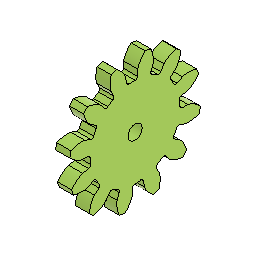
03 Engranaje (para servomotor) (Autodesk Fusion 360 design; units mm, degrees)
Autodesk Fusion 360 part; units mm, degrees
(part 1 of 2)
sketch "Boceto1" plane through (0, 0, 0) normal (0, 0, 1) x (1, 0, 0)
  circle A0 centre (0, 0) radius 9.5
  circle A1 centre (0, 0) radius 0.5
extrude "Extruir1" add sketch "Boceto1" along normal blind 3
sketch "Boceto2" plane through (0, 0, 0) normal (0, 0, 1) x (1, 0, 0)
  spline S0 degree 5 poles (11.1567, -1.6383) (11.1647, -1.6395) (11.1807, -1.6416) (11.2048, -1.6439) (11.237, -1.6456) (11.2774, -1.6458) (11.318, -1.6445) (11.3587, -1.6423) (11.3994, -1.6396) (11.4401, -1.6366) (11.4809, -1.6333) (11.5218, -1.6295) (11.5626, -1.625) (11.6035, -1.6199) (11.6445, -1.614) (11.6854, -1.6075) (11.7264, -1.6005) (11.7674, -1.5929) (11.8084, -1.585) (11.8494, -1.5766) (11.8905, -1.5678) (11.9315, -1.5587) (11.9725, -1.5491) (12.0135, -1.539) (12.0545, -1.5285) (12.0956, -1.5175) (12.1366, -1.5062) (12.1776, -1.4944) (12.2186, -1.4823) (12.2595, -1.4698) (12.3005, -1.4569) (12.3414, -1.4437) (12.3824, -1.4301) (12.4233, -1.4161) (12.4641, -1.4018) (12.505, -1.3871) (12.5458, -1.372) (12.5866, -1.3566) (12.6274, -1.3409) (12.6681, -1.3248) (12.7088, -1.3084) (12.7495, -1.2917) (12.7902, -1.2746) (12.8308, -1.2572) (12.8713, -1.2395) (12.9119, -1.2215) (12.9523, -1.2031) (12.9928, -1.1844) (13.0332, -1.1654) (13.0735, -1.1461) (13.1138, -1.1265) (13.1541, -1.1066) (13.1943, -1.0863) (13.2345, -1.0658) (13.2746, -1.045) (13.3146, -1.0239) (13.3546, -1.0024) (13.3946, -0.9807) (13.4344, -0.9587) (13.4743, -0.9364) (13.514, -0.9138) (13.5538, -0.8909) (13.5934, -0.8678) (13.633, -0.8443) (13.6725, -0.8206) (13.712, -0.7966) (13.7514, -0.7723) (13.7907, -0.7477) (13.8299, -0.7229) (13.8691, -0.6978) (13.9082, -0.6724) (13.9395, -0.6518) (13.9629, -0.6363) (13.9784, -0.6259) (13.9862, -0.6207) knots 0 0 0 0 0 0 0.01428571 0.02857143 0.04285714 0.05714286 0.07142857 0.08571429 0.1 0.11428571 0.12857143 0.14285714 0.15714286 0.17142857 0.18571429 0.2 0.21428571 0.22857143 0.24285714 0.25714286 0.27142857 0.28571429 0.3 0.31428571 0.32857143 0.34285714 0.35714286 0.37142857 0.38571429 0.4 0.41428571 0.42857143 0.44285714 0.45714286 0.47142857 0.48571429 0.5 0.51428571 0.52857143 0.54285714 0.55714286 0.57142857 0.58571429 0.6 0.61428571 0.62857143 0.64285714 0.65714286 0.67142857 0.68571429 0.7 0.71428571 0.72857143 0.74285714 0.75714286 0.77142857 0.78571429 0.8 0.81428571 0.82857143 0.84285714 0.85714286 0.87142857 0.88571429 0.9 0.91428571 0.92857143 0.94285714 0.95714286 0.97142857 0.98571429 1 1 1 1 1 1
  spline S1 degree 5 poles (11.1567, 1.6383) (11.1647, 1.6395) (11.1807, 1.6416) (11.2048, 1.6439) (11.237, 1.6456) (11.2774, 1.6458) (11.318, 1.6445) (11.3587, 1.6423) (11.3994, 1.6396) (11.4401, 1.6366) (11.4809, 1.6333) (11.5218, 1.6295) (11.5626, 1.625) (11.6035, 1.6199) (11.6445, 1.614) (11.6854, 1.6075) (11.7264, 1.6005) (11.7674, 1.5929) (11.8084, 1.585) (11.8494, 1.5766) (11.8905, 1.5678) (11.9315, 1.5587) (11.9725, 1.5491) (12.0135, 1.539) (12.0545, 1.5285) (12.0956, 1.5175) (12.1366, 1.5062) (12.1776, 1.4944) (12.2186, 1.4823) (12.2595, 1.4698) (12.3005, 1.4569) (12.3414, 1.4437) (12.3824, 1.4301) (12.4233, 1.4161) (12.4641, 1.4018) (12.505, 1.3871) (12.5458, 1.372) (12.5866, 1.3566) (12.6274, 1.3409) (12.6681, 1.3248) (12.7088, 1.3084) (12.7495, 1.2917) (12.7902, 1.2746) (12.8308, 1.2572) (12.8713, 1.2395) (12.9119, 1.2215) (12.9523, 1.2031) (12.9928, 1.1844) (13.0332, 1.1654) (13.0735, 1.1461) (13.1138, 1.1265) (13.1541, 1.1066) (13.1943, 1.0863) (13.2345, 1.0658) (13.2746, 1.045) (13.3146, 1.0239) (13.3546, 1.0024) (13.3946, 0.9807) (13.4344, 0.9587) (13.4743, 0.9364) (13.514, 0.9138) (13.5538, 0.8909) (13.5934, 0.8678) (13.633, 0.8443) (13.6725, 0.8206) (13.712, 0.7966) (13.7514, 0.7723) (13.7907, 0.7477) (13.8299, 0.7229) (13.8691, 0.6978) (13.9082, 0.6724) (13.9395, 0.6518) (13.9629, 0.6363) (13.9784, 0.6259) (13.9862, 0.6207) knots 0 0 0 0 0 0 0.01428571 0.02857143 0.04285714 0.05714286 0.07142857 0.08571429 0.1 0.11428571 0.12857143 0.14285714 0.15714286 0.17142857 0.18571429 0.2 0.21428571 0.22857143 0.24285714 0.25714286 0.27142857 0.28571429 0.3 0.31428571 0.32857143 0.34285714 0.35714286 0.37142857 0.38571429 0.4 0.41428571 0.42857143 0.44285714 0.45714286 0.47142857 0.48571429 0.5 0.51428571 0.52857143 0.54285714 0.55714286 0.57142857 0.58571429 0.6 0.61428571 0.62857143 0.64285714 0.65714286 0.67142857 0.68571429 0.7 0.71428571 0.72857143 0.74285714 0.75714286 0.77142857 0.78571429 0.8 0.81428571 0.82857143 0.84285714 0.85714286 0.87142857 0.88571429 0.9 0.91428571 0.92857143 0.94285714 0.95714286 0.97142857 0.98571429 1 1 1 1 1 1
  arc A0 (13.9862, -0.6207) -> (13.9862, 0.6207) centre (0, 0) ccw
  line L0 (9.3893, -1.3802) -> (11.1567, -1.6383)
  line L1 (9.3893, 1.3802) -> (11.1567, 1.6383)
  line L2 (9.3893, -1.3802) -> (9.3893, 1.3802)
  point P0 (11.3527, -1.6425)
  point P1 (11.5515, -1.6261)
  point P2 (11.7521, -1.5957)
  point P3 (11.954, -1.5533)
  point P4 (12.1568, -1.5003)
  point P5 (12.3603, -1.4374)
  point P6 (12.5642, -1.3651)
  point P7 (12.7683, -1.2838)
  point P8 (12.9724, -1.1938)
  point P9 (13.1764, -1.0953)
  point P10 (13.3799, -0.9887)
  point P11 (13.5828, -0.8739)
  point P12 (13.785, -0.7512)
  point P13 (11.3527, 1.6425)
  point P14 (11.5515, 1.6261)
  point P15 (11.7521, 1.5957)
  point P16 (11.954, 1.5533)
  point P17 (12.1568, 1.5003)
  point P18 (12.3603, 1.4374)
  point P19 (12.5642, 1.3651)
  point P20 (12.7683, 1.2838)
  point P21 (12.9724, 1.1938)
  point P22 (13.1764, 1.0953)
  point P23 (13.3799, 0.9887)
  point P24 (13.5828, 0.8739)
  point P25 (13.785, 0.7512)
extrude "Extruir2" add sketch "Boceto2" along normal blind 3
fillet "Empalme1" radius 0.5 2 edges at (9.399, -1.3817, 1.5) (9.399, 1.3817, 1.5)
pattern_circular "Patrón C1" count 12 over 360 about axis through (0, 0, 0) along (0, 0, 1) of "Extruir2", "Empalme1"
sketch "Boceto3" plane through (0, 0, 0) normal (0, 0, 1) x (1, 0, 0)
  circle A0 centre (0, 0) radius 12 construction
move_body "Desplazar1" bodies 1 to x (0.660356, 0.750952, 0) y (-0.750952, 0.660356, 0) z (0, 0, 1) at (0, 0, 0)
move_body "Desplazar2" bodies 1 to x (0, 0, -1) y (0, 1, 0) z (1, 0, 0) at (0, 0, 0)
move_body "Desplazar3" bodies 1 to x (1, 0, 0) y (0, 1, 0) z (0, 0, 1) at (0, 47.5478, 13.9934)
sketch "Boceto4" plane through (0, 0, 0) normal (-1, 0, 0) x (0, -1, 0)
  circle A0 centre (-47.5478, 13.9934) radius 0.5
  arc A1 (-47.0309, 4.0198) -> (-47.5311, 4.4934) centre (-47.5302, 3.9934) ccw
  line L0 (-47.0309, 4.0198) -> (-46.963, 2.7323)
  spline S0 degree 5 poles (-46.963, 2.7323) (-46.9625, 2.7242) (-46.9614, 2.7081) (-46.959, 2.684) (-46.9543, 2.6521) (-46.9465, 2.6124) (-46.9373, 2.5729) (-46.9272, 2.5335) (-46.9166, 2.494) (-46.9056, 2.4547) (-46.8943, 2.4153) (-46.8826, 2.3761) (-46.8702, 2.3369) (-46.8571, 2.2978) (-46.8433, 2.2588) (-46.8289, 2.2199) (-46.8139, 2.1811) (-46.7985, 2.1424) (-46.7826, 2.1037) (-46.7664, 2.0651) (-46.7497, 2.0266) (-46.7327, 1.9882) (-46.7152, 1.9499) (-46.6973, 1.9116) (-46.6789, 1.8735) (-46.6601, 1.8354) (-46.6409, 1.7974) (-46.6213, 1.7595) (-46.6014, 1.7217) (-46.5811, 1.684) (-46.5604, 1.6464) (-46.5394, 1.6088) (-46.5181, 1.5714) (-46.4963, 1.534) (-46.4742, 1.4967) (-46.4518, 1.4596) (-46.429, 1.4225) (-46.4059, 1.3855) (-46.3825, 1.3486) (-46.3587, 1.3118) (-46.3346, 1.2751) (-46.3102, 1.2385) (-46.2855, 1.202) (-46.2605, 1.1656) (-46.2351, 1.1294) (-46.2095, 1.0932) (-46.1835, 1.0571) (-46.1573, 1.0211) (-46.1307, 0.9852) (-46.1039, 0.9494) (-46.0767, 0.9138) (-46.0493, 0.8782) (-46.0215, 0.8428) (-45.9935, 0.8074) (-45.9652, 0.7722) (-45.9366, 0.7371) (-45.9078, 0.702) (-45.8786, 0.6671) (-45.8492, 0.6324) (-45.8195, 0.5977) (-45.7896, 0.5631) (-45.7593, 0.5287) (-45.7288, 0.4944) (-45.698, 0.4601) (-45.667, 0.4261) (-45.6357, 0.3921) (-45.6042, 0.3582) (-45.5724, 0.3245) (-45.5403, 0.2909) (-45.508, 0.2574) (-45.4754, 0.224) (-45.4491, 0.1974) (-45.4293, 0.1776) (-45.416, 0.1643) (-45.4094, 0.1577) knots 0 0 0 0 0 0 0.01428571 0.02857143 0.04285714 0.05714286 0.07142857 0.08571429 0.1 0.11428571 0.12857143 0.14285714 0.15714286 0.17142857 0.18571429 0.2 0.21428571 0.22857143 0.24285714 0.25714286 0.27142857 0.28571429 0.3 0.31428571 0.32857143 0.34285714 0.35714286 0.37142857 0.38571429 0.4 0.41428571 0.42857143 0.44285714 0.45714286 0.47142857 0.48571429 0.5 0.51428571 0.52857143 0.54285714 0.55714286 0.57142857 0.58571429 0.6 0.61428571 0.62857143 0.64285714 0.65714286 0.67142857 0.68571429 0.7 0.71428571 0.72857143 0.74285714 0.75714286 0.77142857 0.78571429 0.8 0.81428571 0.82857143 0.84285714 0.85714286 0.87142857 0.88571429 0.9 0.91428571 0.92857143 0.94285714 0.95714286 0.97142857 0.98571429 1 1 1 1 1 1
  arc A2 (-45.4094, 0.1577) -> (-44.1922, 0.4015) centre (-47.5478, 13.9934) ccw
  spline S1 degree 5 poles (-43.7502, 3.3759) (-43.7474, 3.3682) (-43.7423, 3.3529) (-43.7352, 3.3298) (-43.7272, 3.2985) (-43.7191, 3.2589) (-43.7124, 3.2189) (-43.7066, 3.1786) (-43.7012, 3.1381) (-43.6961, 3.0976) (-43.6914, 3.0569) (-43.6871, 3.0161) (-43.6834, 2.9752) (-43.6805, 2.9341) (-43.6782, 2.8928) (-43.6765, 2.8513) (-43.6754, 2.8098) (-43.6747, 2.7681) (-43.6745, 2.7263) (-43.6746, 2.6845) (-43.6751, 2.6425) (-43.6761, 2.6005) (-43.6774, 2.5584) (-43.6792, 2.5162) (-43.6815, 2.4739) (-43.6842, 2.4315) (-43.6873, 2.3891) (-43.6907, 2.3466) (-43.6946, 2.304) (-43.6988, 2.2614) (-43.7033, 2.2187) (-43.7083, 2.1759) (-43.7136, 2.1331) (-43.7192, 2.0903) (-43.7253, 2.0474) (-43.7317, 2.0044) (-43.7384, 1.9614) (-43.7455, 1.9184) (-43.7529, 1.8753) (-43.7606, 1.8322) (-43.7687, 1.7891) (-43.7772, 1.7459) (-43.7859, 1.7027) (-43.795, 1.6595) (-43.8044, 1.6163) (-43.8142, 1.573) (-43.8242, 1.5297) (-43.8346, 1.4864) (-43.8453, 1.443) (-43.8563, 1.3997) (-43.8676, 1.3563) (-43.8792, 1.3129) (-43.8912, 1.2695) (-43.9034, 1.2261) (-43.9159, 1.1827) (-43.9288, 1.1392) (-43.9419, 1.0958) (-43.9554, 1.0524) (-43.9691, 1.009) (-43.9832, 0.9655) (-43.9975, 0.9221) (-44.0122, 0.8787) (-44.0271, 0.8352) (-44.0423, 0.7918) (-44.0578, 0.7484) (-44.0736, 0.705) (-44.0897, 0.6616) (-44.1061, 0.6182) (-44.1227, 0.5748) (-44.1396, 0.5315) (-44.1569, 0.4882) (-44.1708, 0.4535) (-44.1815, 0.4275) (-44.1886, 0.4102) (-44.1922, 0.4015) knots 0 0 0 0 0 0 0.01428571 0.02857143 0.04285714 0.05714286 0.07142857 0.08571429 0.1 0.11428571 0.12857143 0.14285714 0.15714286 0.17142857 0.18571429 0.2 0.21428571 0.22857143 0.24285714 0.25714286 0.27142857 0.28571429 0.3 0.31428571 0.32857143 0.34285714 0.35714286 0.37142857 0.38571429 0.4 0.41428571 0.42857143 0.44285714 0.45714286 0.47142857 0.48571429 0.5 0.51428571 0.52857143 0.54285714 0.55714286 0.57142857 0.58571429 0.6 0.61428571 0.62857143 0.64285714 0.65714286 0.67142857 0.68571429 0.7 0.71428571 0.72857143 0.74285714 0.75714286 0.77142857 0.78571429 0.8 0.81428571 0.82857143 0.84285714 0.85714286 0.87142857 0.88571429 0.9 0.91428571 0.92857143 0.94285714 0.95714286 0.97142857 0.98571429 1 1 1 1 1 1
  line L1 (-43.7502, 3.3759) -> (-44.1834, 4.5902)
  arc A3 (-43.9042, 5.2199) -> (-44.1834, 4.5902) centre (-43.7125, 4.7582) ccw
  arc A4 (-43.9042, 5.2199) -> (-42.7833, 5.7746) centre (-47.5478, 13.9934) ccw
  arc A5 (-42.1133, 5.6145) -> (-42.7833, 5.7746) centre (-42.5325, 5.342) ccw
  line L2 (-42.1133, 5.6145) -> (-41.4107, 4.5334)
  spline S2 degree 5 poles (-41.4107, 4.5334) (-41.4063, 4.5267) (-41.3973, 4.5133) (-41.3832, 4.4936) (-41.3632, 4.4683) (-41.3366, 4.4378) (-41.3088, 4.4082) (-41.2803, 4.3791) (-41.2515, 4.3503) (-41.2223, 4.3217) (-41.1928, 4.2933) (-41.163, 4.2651) (-41.1327, 4.2374) (-41.1018, 4.21) (-41.0704, 4.1832) (-41.0385, 4.1567) (-41.0061, 4.1306) (-40.9733, 4.1048) (-40.9403, 4.0792) (-40.9069, 4.0539) (-40.8733, 4.0289) (-40.8393, 4.0042) (-40.805, 3.9797) (-40.7703, 3.9556) (-40.7353, 3.9317) (-40.7, 3.9081) (-40.6644, 3.8848) (-40.6285, 3.8618) (-40.5923, 3.839) (-40.5559, 3.8165) (-40.5192, 3.7942) (-40.4822, 3.7722) (-40.445, 3.7505) (-40.4075, 3.729) (-40.3697, 3.7078) (-40.3317, 3.6868) (-40.2934, 3.6661) (-40.2549, 3.6456) (-40.2162, 3.6254) (-40.1772, 3.6054) (-40.138, 3.5857) (-40.0986, 3.5662) (-40.0589, 3.5469) (-40.0191, 3.5279) (-39.979, 3.5092) (-39.9387, 3.4906) (-39.8981, 3.4724) (-39.8574, 3.4543) (-39.8165, 3.4365) (-39.7753, 3.419) (-39.734, 3.4017) (-39.6924, 3.3846) (-39.6507, 3.3678) (-39.6087, 3.3512) (-39.5666, 3.3348) (-39.5243, 3.3187) (-39.4818, 3.3028) (-39.4391, 3.2871) (-39.3962, 3.2717) (-39.3532, 3.2565) (-39.31, 3.2416) (-39.2666, 3.2269) (-39.223, 3.2124) (-39.1792, 3.1981) (-39.1353, 3.1841) (-39.0912, 3.1704) (-39.047, 3.1568) (-39.0026, 3.1435) (-38.958, 3.1304) (-38.9132, 3.1176) (-38.8683, 3.105) (-38.8323, 3.0951) (-38.8052, 3.0878) (-38.7871, 3.083) (-38.778, 3.0806) knots 0 0 0 0 0 0 0.01428571 0.02857143 0.04285714 0.05714286 0.07142857 0.08571429 0.1 0.11428571 0.12857143 0.14285714 0.15714286 0.17142857 0.18571429 0.2 0.21428571 0.22857143 0.24285714 0.25714286 0.27142857 0.28571429 0.3 0.31428571 0.32857143 0.34285714 0.35714286 0.37142857 0.38571429 0.4 0.41428571 0.42857143 0.44285714 0.45714286 0.47142857 0.48571429 0.5 0.51428571 0.52857143 0.54285714 0.55714286 0.57142857 0.58571429 0.6 0.61428571 0.62857143 0.64285714 0.65714286 0.67142857 0.68571429 0.7 0.71428571 0.72857143 0.74285714 0.75714286 0.77142857 0.78571429 0.8 0.81428571 0.82857143 0.84285714 0.85714286 0.87142857 0.88571429 0.9 0.91428571 0.92857143 0.94285714 0.95714286 0.97142857 0.98571429 1 1 1 1 1 1
  arc A6 (-38.778, 3.0806) -> (-37.8458, 3.9003) centre (-47.5478, 13.9934) ccw
  spline S3 degree 5 poles (-38.9502, 6.6972) (-38.944, 6.6919) (-38.9319, 6.6813) (-38.9142, 6.6648) (-38.8916, 6.6417) (-38.8648, 6.6114) (-38.839, 6.5801) (-38.8138, 6.5481) (-38.7889, 6.5158) (-38.7642, 6.4832) (-38.7398, 6.4503) (-38.7157, 6.4172) (-38.6921, 6.3835) (-38.6689, 6.3494) (-38.6463, 6.3148) (-38.6241, 6.2798) (-38.6023, 6.2443) (-38.5809, 6.2086) (-38.5598, 6.1725) (-38.539, 6.1362) (-38.5185, 6.0996) (-38.4983, 6.0627) (-38.4784, 6.0256) (-38.4589, 5.9881) (-38.4397, 5.9504) (-38.4209, 5.9123) (-38.4023, 5.874) (-38.384, 5.8355) (-38.3661, 5.7967) (-38.3484, 5.7577) (-38.331, 5.7184) (-38.3139, 5.6789) (-38.2971, 5.6392) (-38.2806, 5.5993) (-38.2644, 5.5591) (-38.2484, 5.5187) (-38.2328, 5.4781) (-38.2174, 5.4373) (-38.2023, 5.3963) (-38.1874, 5.3551) (-38.1729, 5.3137) (-38.1586, 5.2721) (-38.1446, 5.2303) (-38.1308, 5.1884) (-38.1174, 5.1462) (-38.1041, 5.1038) (-38.0912, 5.0613) (-38.0785, 5.0186) (-38.0661, 4.9757) (-38.054, 4.9327) (-38.0421, 4.8895) (-38.0305, 4.8461) (-38.0191, 4.8025) (-38.008, 4.7588) (-37.9971, 4.7149) (-37.9866, 4.6709) (-37.9762, 4.6267) (-37.9662, 4.5824) (-37.9564, 4.5379) (-37.9468, 4.4932) (-37.9375, 4.4485) (-37.9285, 4.4035) (-37.9197, 4.3585) (-37.9111, 4.3132) (-37.9029, 4.2679) (-37.8948, 4.2224) (-37.8871, 4.1768) (-37.8796, 4.131) (-37.8723, 4.0852) (-37.8653, 4.0391) (-37.8585, 3.993) (-37.8533, 3.956) (-37.8495, 3.9282) (-37.847, 3.9096) (-37.8458, 3.9003) knots 0 0 0 0 0 0 0.01428571 0.02857143 0.04285714 0.05714286 0.07142857 0.08571429 0.1 0.11428571 0.12857143 0.14285714 0.15714286 0.17142857 0.18571429 0.2 0.21428571 0.22857143 0.24285714 0.25714286 0.27142857 0.28571429 0.3 0.31428571 0.32857143 0.34285714 0.35714286 0.37142857 0.38571429 0.4 0.41428571 0.42857143 0.44285714 0.45714286 0.47142857 0.48571429 0.5 0.51428571 0.52857143 0.54285714 0.55714286 0.57142857 0.58571429 0.6 0.61428571 0.62857143 0.64285714 0.65714286 0.67142857 0.68571429 0.7 0.71428571 0.72857143 0.74285714 0.75714286 0.77142857 0.78571429 0.8 0.81428571 0.82857143 0.84285714 0.85714286 0.87142857 0.88571429 0.9 0.91428571 0.92857143 0.94285714 0.95714286 0.97142857 0.98571429 1 1 1 1 1 1
  line L3 (-38.9502, 6.6972) -> (-39.9325, 7.5322)
  arc A7 (-40.0056, 8.2172) -> (-39.9325, 7.5322) centre (-39.6087, 7.9131) ccw
  arc A8 (-40.0056, 8.2172) -> (-39.3122, 9.258) centre (-47.5478, 13.9934) ccw
  arc A9 (-38.6519, 9.4543) -> (-39.3122, 9.258) centre (-38.8788, 9.0087) ccw
  line L4 (-38.6519, 9.4543) -> (-37.503, 8.8694)
  spline S4 degree 5 poles (-37.503, 8.8694) (-37.4958, 8.8657) (-37.4813, 8.8586) (-37.4592, 8.8487) (-37.4292, 8.8367) (-37.3909, 8.8237) (-37.3521, 8.8119) (-37.3129, 8.8009) (-37.2734, 8.7904) (-37.2339, 8.7802) (-37.1942, 8.7703) (-37.1543, 8.7609) (-37.1141, 8.752) (-37.0737, 8.7438) (-37.0331, 8.7362) (-36.9922, 8.7292) (-36.9511, 8.7228) (-36.9098, 8.7168) (-36.8684, 8.7112) (-36.8269, 8.706) (-36.7852, 8.7012) (-36.7434, 8.6967) (-36.7015, 8.6927) (-36.6594, 8.6891) (-36.6172, 8.686) (-36.5748, 8.6832) (-36.5323, 8.6808) (-36.4897, 8.6788) (-36.447, 8.6772) (-36.4042, 8.6759) (-36.3613, 8.675) (-36.3182, 8.6744) (-36.2751, 8.6742) (-36.2319, 8.6743) (-36.1886, 8.6748) (-36.1452, 8.6757) (-36.1017, 8.6769) (-36.0581, 8.6784) (-36.0144, 8.6802) (-35.9707, 8.6824) (-35.9269, 8.6849) (-35.883, 8.6878) (-35.839, 8.6909) (-35.795, 8.6944) (-35.7509, 8.6982) (-35.7067, 8.7023) (-35.6625, 8.7068) (-35.6182, 8.7115) (-35.5738, 8.7166) (-35.5294, 8.722) (-35.485, 8.7276) (-35.4404, 8.7336) (-35.3959, 8.7399) (-35.3512, 8.7465) (-35.3066, 8.7534) (-35.2619, 8.7606) (-35.2171, 8.7681) (-35.1723, 8.7759) (-35.1275, 8.7839) (-35.0826, 8.7923) (-35.0377, 8.801) (-34.9928, 8.8099) (-34.9478, 8.8192) (-34.9028, 8.8287) (-34.8577, 8.8386) (-34.8127, 8.8487) (-34.7676, 8.8591) (-34.7225, 8.8698) (-34.6773, 8.8807) (-34.6321, 8.892) (-34.587, 8.9035) (-34.5508, 8.913) (-34.5237, 8.9202) (-34.5056, 8.925) (-34.4965, 8.9275) knots 0 0 0 0 0 0 0.01428571 0.02857143 0.04285714 0.05714286 0.07142857 0.08571429 0.1 0.11428571 0.12857143 0.14285714 0.15714286 0.17142857 0.18571429 0.2 0.21428571 0.22857143 0.24285714 0.25714286 0.27142857 0.28571429 0.3 0.31428571 0.32857143 0.34285714 0.35714286 0.37142857 0.38571429 0.4 0.41428571 0.42857143 0.44285714 0.45714286 0.47142857 0.48571429 0.5 0.51428571 0.52857143 0.54285714 0.55714286 0.57142857 0.58571429 0.6 0.61428571 0.62857143 0.64285714 0.65714286 0.67142857 0.68571429 0.7 0.71428571 0.72857143 0.74285714 0.75714286 0.77142857 0.78571429 0.8 0.81428571 0.82857143 0.84285714 0.85714286 0.87142857 0.88571429 0.9 0.91428571 0.92857143 0.94285714 0.95714286 0.97142857 0.98571429 1 1 1 1 1 1
  arc A10 (-34.4965, 8.9275) -> (-34.0991, 10.1035) centre (-47.5478, 13.9934) ccw
  spline S5 degree 5 poles (-36.4539, 11.9735) (-36.446, 11.9721) (-36.4301, 11.9689) (-36.4065, 11.9634) (-36.3755, 11.9547) (-36.3371, 11.9419) (-36.2991, 11.9277) (-36.2613, 11.9126) (-36.2235, 11.8971) (-36.1859, 11.8812) (-36.1483, 11.8649) (-36.1109, 11.8482) (-36.0736, 11.831) (-36.0365, 11.813) (-35.9996, 11.7943) (-35.9628, 11.7751) (-35.9263, 11.7552) (-35.8898, 11.735) (-35.8535, 11.7143) (-35.8174, 11.6933) (-35.7813, 11.6718) (-35.7454, 11.65) (-35.7096, 11.6278) (-35.6739, 11.6051) (-35.6384, 11.582) (-35.6031, 11.5585) (-35.5679, 11.5346) (-35.5328, 11.5103) (-35.4978, 11.4857) (-35.463, 11.4608) (-35.4283, 11.4355) (-35.3938, 11.4098) (-35.3594, 11.3838) (-35.3251, 11.3575) (-35.291, 11.3308) (-35.257, 11.3038) (-35.2231, 11.2765) (-35.1894, 11.2489) (-35.1558, 11.2209) (-35.1223, 11.1926) (-35.089, 11.1641) (-35.0559, 11.1352) (-35.0228, 11.106) (-34.9899, 11.0765) (-34.9572, 11.0467) (-34.9246, 11.0167) (-34.8921, 10.9863) (-34.8598, 10.9557) (-34.8276, 10.9247) (-34.7955, 10.8935) (-34.7636, 10.862) (-34.7319, 10.8303) (-34.7002, 10.7982) (-34.6688, 10.7659) (-34.6374, 10.7333) (-34.6063, 10.7005) (-34.5752, 10.6674) (-34.5443, 10.634) (-34.5136, 10.6004) (-34.483, 10.5665) (-34.4526, 10.5324) (-34.4223, 10.498) (-34.3921, 10.4634) (-34.3621, 10.4285) (-34.3323, 10.3933) (-34.3026, 10.358) (-34.2731, 10.3223) (-34.2437, 10.2865) (-34.2144, 10.2504) (-34.1854, 10.214) (-34.1564, 10.1775) (-34.1334, 10.148) (-34.1162, 10.1258) (-34.1048, 10.111) (-34.0991, 10.1035) knots 0 0 0 0 0 0 0.01428571 0.02857143 0.04285714 0.05714286 0.07142857 0.08571429 0.1 0.11428571 0.12857143 0.14285714 0.15714286 0.17142857 0.18571429 0.2 0.21428571 0.22857143 0.24285714 0.25714286 0.27142857 0.28571429 0.3 0.31428571 0.32857143 0.34285714 0.35714286 0.37142857 0.38571429 0.4 0.41428571 0.42857143 0.44285714 0.45714286 0.47142857 0.48571429 0.5 0.51428571 0.52857143 0.54285714 0.55714286 0.57142857 0.58571429 0.6 0.61428571 0.62857143 0.64285714 0.65714286 0.67142857 0.68571429 0.7 0.71428571 0.72857143 0.74285714 0.75714286 0.77142857 0.78571429 0.8 0.81428571 0.82857143 0.84285714 0.85714286 0.87142857 0.88571429 0.9 0.91428571 0.92857143 0.94285714 0.95714286 0.97142857 0.98571429 1 1 1 1 1 1
  line L5 (-36.4539, 11.9735) -> (-37.7221, 12.2055)
  arc A11 (-38.128, 12.7621) -> (-37.7221, 12.2055) centre (-37.6322, 12.6973) ccw
  arc A12 (-38.128, 12.7621) -> (-38.0478, 14.0102) centre (-47.5478, 13.9934) ccw
  arc A13 (-37.5742, 14.5104) -> (-38.0478, 14.0102) centre (-37.5478, 14.0111) ccw
  line L6 (-37.5742, 14.5104) -> (-36.2867, 14.5783)
  spline S6 degree 5 poles (-36.2867, 14.5783) (-36.2786, 14.5787) (-36.2625, 14.5798) (-36.2384, 14.5822) (-36.2065, 14.5869) (-36.1668, 14.5947) (-36.1273, 14.604) (-36.0879, 14.6141) (-36.0484, 14.6247) (-36.0091, 14.6356) (-35.9697, 14.6469) (-35.9305, 14.6587) (-35.8913, 14.6711) (-35.8522, 14.6841) (-35.8132, 14.6979) (-35.7743, 14.7123) (-35.7355, 14.7273) (-35.6968, 14.7428) (-35.6581, 14.7586) (-35.6195, 14.7749) (-35.581, 14.7915) (-35.5426, 14.8086) (-35.5043, 14.8261) (-35.466, 14.844) (-35.4279, 14.8624) (-35.3898, 14.8811) (-35.3518, 14.9003) (-35.3139, 14.9199) (-35.2761, 14.9398) (-35.2384, 14.9601) (-35.2008, 14.9808) (-35.1632, 15.0018) (-35.1258, 15.0232) (-35.0884, 15.0449) (-35.0511, 15.067) (-35.014, 15.0895) (-34.9769, 15.1122) (-34.9399, 15.1353) (-34.903, 15.1588) (-34.8662, 15.1825) (-34.8295, 15.2066) (-34.7929, 15.231) (-34.7564, 15.2557) (-34.72, 15.2808) (-34.6838, 15.3061) (-34.6476, 15.3318) (-34.6115, 15.3577) (-34.5755, 15.384) (-34.5396, 15.4105) (-34.5038, 15.4374) (-34.4682, 15.4645) (-34.4326, 15.492) (-34.3972, 15.5197) (-34.3618, 15.5477) (-34.3266, 15.576) (-34.2915, 15.6046) (-34.2564, 15.6335) (-34.2215, 15.6626) (-34.1868, 15.692) (-34.1521, 15.7217) (-34.1175, 15.7517) (-34.0831, 15.7819) (-34.0488, 15.8124) (-34.0145, 15.8432) (-33.9805, 15.8742) (-33.9465, 15.9055) (-33.9126, 15.9371) (-33.8789, 15.9689) (-33.8453, 16.001) (-33.8118, 16.0333) (-33.7784, 16.0659) (-33.7518, 16.0921) (-33.732, 16.1119) (-33.7187, 16.1252) (-33.7121, 16.1318) knots 0 0 0 0 0 0 0.01428571 0.02857143 0.04285714 0.05714286 0.07142857 0.08571429 0.1 0.11428571 0.12857143 0.14285714 0.15714286 0.17142857 0.18571429 0.2 0.21428571 0.22857143 0.24285714 0.25714286 0.27142857 0.28571429 0.3 0.31428571 0.32857143 0.34285714 0.35714286 0.37142857 0.38571429 0.4 0.41428571 0.42857143 0.44285714 0.45714286 0.47142857 0.48571429 0.5 0.51428571 0.52857143 0.54285714 0.55714286 0.57142857 0.58571429 0.6 0.61428571 0.62857143 0.64285714 0.65714286 0.67142857 0.68571429 0.7 0.71428571 0.72857143 0.74285714 0.75714286 0.77142857 0.78571429 0.8 0.81428571 0.82857143 0.84285714 0.85714286 0.87142857 0.88571429 0.9 0.91428571 0.92857143 0.94285714 0.95714286 0.97142857 0.98571429 1 1 1 1 1 1
  arc A14 (-33.7121, 16.1318) -> (-33.9559, 17.3491) centre (-47.5478, 13.9934) ccw
  spline S7 degree 5 poles (-36.9303, 17.7911) (-36.9226, 17.7938) (-36.9073, 17.799) (-36.8842, 17.806) (-36.8529, 17.814) (-36.8133, 17.8221) (-36.7733, 17.8288) (-36.733, 17.8347) (-36.6925, 17.8401) (-36.652, 17.8451) (-36.6113, 17.8499) (-36.5705, 17.8541) (-36.5296, 17.8578) (-36.4885, 17.8608) (-36.4472, 17.8631) (-36.4058, 17.8648) (-36.3642, 17.8659) (-36.3225, 17.8665) (-36.2807, 17.8668) (-36.2389, 17.8667) (-36.1969, 17.8661) (-36.1549, 17.8652) (-36.1128, 17.8638) (-36.0706, 17.862) (-36.0283, 17.8597) (-35.9859, 17.8571) (-35.9435, 17.854) (-35.901, 17.8505) (-35.8584, 17.8467) (-35.8158, 17.8425) (-35.7731, 17.8379) (-35.7303, 17.833) (-35.6875, 17.8277) (-35.6447, 17.822) (-35.6018, 17.816) (-35.5588, 17.8096) (-35.5158, 17.8029) (-35.4728, 17.7958) (-35.4298, 17.7884) (-35.3866, 17.7806) (-35.3435, 17.7725) (-35.3003, 17.7641) (-35.2571, 17.7553) (-35.2139, 17.7462) (-35.1707, 17.7368) (-35.1274, 17.7271) (-35.0841, 17.717) (-35.0408, 17.7067) (-34.9974, 17.696) (-34.9541, 17.685) (-34.9107, 17.6737) (-34.8673, 17.662) (-34.8239, 17.6501) (-34.7805, 17.6379) (-34.7371, 17.6253) (-34.6936, 17.6125) (-34.6502, 17.5993) (-34.6068, 17.5859) (-34.5634, 17.5721) (-34.5199, 17.5581) (-34.4765, 17.5437) (-34.4331, 17.5291) (-34.3896, 17.5142) (-34.3462, 17.4989) (-34.3028, 17.4834) (-34.2594, 17.4676) (-34.216, 17.4516) (-34.1726, 17.4352) (-34.1292, 17.4185) (-34.0859, 17.4016) (-34.0426, 17.3844) (-34.0079, 17.3704) (-33.9819, 17.3598) (-33.9646, 17.3526) (-33.9559, 17.3491) knots 0 0 0 0 0 0 0.01428571 0.02857143 0.04285714 0.05714286 0.07142857 0.08571429 0.1 0.11428571 0.12857143 0.14285714 0.15714286 0.17142857 0.18571429 0.2 0.21428571 0.22857143 0.24285714 0.25714286 0.27142857 0.28571429 0.3 0.31428571 0.32857143 0.34285714 0.35714286 0.37142857 0.38571429 0.4 0.41428571 0.42857143 0.44285714 0.45714286 0.47142857 0.48571429 0.5 0.51428571 0.52857143 0.54285714 0.55714286 0.57142857 0.58571429 0.6 0.61428571 0.62857143 0.64285714 0.65714286 0.67142857 0.68571429 0.7 0.71428571 0.72857143 0.74285714 0.75714286 0.77142857 0.78571429 0.8 0.81428571 0.82857143 0.84285714 0.85714286 0.87142857 0.88571429 0.9 0.91428571 0.92857143 0.94285714 0.95714286 0.97142857 0.98571429 1 1 1 1 1 1
  line L7 (-36.9303, 17.7911) -> (-38.1446, 17.3579)
  arc A15 (-38.7743, 17.637) -> (-38.1446, 17.3579) centre (-38.3126, 17.8288) ccw
  arc A16 (-38.7743, 17.637) -> (-39.329, 18.7579) centre (-47.5478, 13.9934) ccw
  arc A17 (-39.1689, 19.428) -> (-39.329, 18.7579) centre (-38.8964, 19.0087) ccw
  line L8 (-39.1689, 19.428) -> (-38.0878, 20.1305)
  spline S8 degree 5 poles (-38.0878, 20.1305) (-38.0811, 20.1349) (-38.0677, 20.1439) (-38.048, 20.158) (-38.0227, 20.1781) (-37.9922, 20.2047) (-37.9626, 20.2324) (-37.9335, 20.2609) (-37.9047, 20.2898) (-37.8761, 20.319) (-37.8477, 20.3484) (-37.8195, 20.3782) (-37.7918, 20.4086) (-37.7644, 20.4394) (-37.7376, 20.4709) (-37.7111, 20.5028) (-37.685, 20.5352) (-37.6592, 20.5679) (-37.6336, 20.601) (-37.6083, 20.6343) (-37.5833, 20.668) (-37.5586, 20.702) (-37.5341, 20.7363) (-37.51, 20.7709) (-37.4861, 20.8059) (-37.4625, 20.8412) (-37.4392, 20.8768) (-37.4162, 20.9127) (-37.3934, 20.9489) (-37.3709, 20.9853) (-37.3486, 21.0221) (-37.3266, 21.059) (-37.3049, 21.0963) (-37.2834, 21.1338) (-37.2622, 21.1715) (-37.2412, 21.2095) (-37.2205, 21.2478) (-37.2, 21.2863) (-37.1798, 21.325) (-37.1598, 21.364) (-37.1401, 21.4032) (-37.1206, 21.4427) (-37.1013, 21.4823) (-37.0823, 21.5222) (-37.0636, 21.5623) (-37.045, 21.6026) (-37.0268, 21.6431) (-37.0087, 21.6839) (-36.9909, 21.7248) (-36.9734, 21.7659) (-36.9561, 21.8073) (-36.939, 21.8488) (-36.9222, 21.8906) (-36.9056, 21.9325) (-36.8892, 21.9746) (-36.8731, 22.0169) (-36.8572, 22.0595) (-36.8415, 22.1021) (-36.8261, 22.145) (-36.8109, 22.1881) (-36.796, 22.2313) (-36.7813, 22.2747) (-36.7668, 22.3183) (-36.7525, 22.362) (-36.7385, 22.4059) (-36.7248, 22.45) (-36.7112, 22.4943) (-36.6979, 22.5387) (-36.6848, 22.5833) (-36.672, 22.628) (-36.6594, 22.6729) (-36.6495, 22.7089) (-36.6422, 22.7361) (-36.6374, 22.7542) (-36.635, 22.7632) knots 0 0 0 0 0 0 0.01428571 0.02857143 0.04285714 0.05714286 0.07142857 0.08571429 0.1 0.11428571 0.12857143 0.14285714 0.15714286 0.17142857 0.18571429 0.2 0.21428571 0.22857143 0.24285714 0.25714286 0.27142857 0.28571429 0.3 0.31428571 0.32857143 0.34285714 0.35714286 0.37142857 0.38571429 0.4 0.41428571 0.42857143 0.44285714 0.45714286 0.47142857 0.48571429 0.5 0.51428571 0.52857143 0.54285714 0.55714286 0.57142857 0.58571429 0.6 0.61428571 0.62857143 0.64285714 0.65714286 0.67142857 0.68571429 0.7 0.71428571 0.72857143 0.74285714 0.75714286 0.77142857 0.78571429 0.8 0.81428571 0.82857143 0.84285714 0.85714286 0.87142857 0.88571429 0.9 0.91428571 0.92857143 0.94285714 0.95714286 0.97142857 0.98571429 1 1 1 1 1 1
  arc A18 (-36.635, 22.7632) -> (-37.4547, 23.6954) centre (-47.5478, 13.9934) ccw
  spline S9 degree 5 poles (-40.2516, 22.5911) (-40.2463, 22.5973) (-40.2357, 22.6094) (-40.2192, 22.6271) (-40.1961, 22.6496) (-40.1658, 22.6764) (-40.1345, 22.7022) (-40.1025, 22.7275) (-40.0702, 22.7524) (-40.0376, 22.777) (-40.0047, 22.8014) (-39.9716, 22.8255) (-39.9379, 22.8492) (-39.9038, 22.8723) (-39.8692, 22.895) (-39.8342, 22.9171) (-39.7987, 22.9389) (-39.763, 22.9603) (-39.7269, 22.9814) (-39.6906, 23.0022) (-39.654, 23.0227) (-39.6171, 23.0429) (-39.58, 23.0628) (-39.5425, 23.0823) (-39.5048, 23.1015) (-39.4667, 23.1204) (-39.4284, 23.139) (-39.3899, 23.1572) (-39.3511, 23.1752) (-39.3121, 23.1928) (-39.2728, 23.2102) (-39.2333, 23.2273) (-39.1936, 23.2441) (-39.1537, 23.2606) (-39.1135, 23.2769) (-39.0731, 23.2928) (-39.0325, 23.3085) (-38.9917, 23.3239) (-38.9507, 23.339) (-38.9095, 23.3538) (-38.8681, 23.3684) (-38.8265, 23.3827) (-38.7847, 23.3967) (-38.7428, 23.4104) (-38.7006, 23.4239) (-38.6582, 23.4371) (-38.6157, 23.45) (-38.573, 23.4627) (-38.5301, 23.4751) (-38.4871, 23.4873) (-38.4439, 23.4992) (-38.4005, 23.5108) (-38.3569, 23.5222) (-38.3132, 23.5333) (-38.2693, 23.5441) (-38.2253, 23.5547) (-38.1811, 23.565) (-38.1368, 23.5751) (-38.0923, 23.5849) (-38.0476, 23.5944) (-38.0029, 23.6037) (-37.9579, 23.6128) (-37.9129, 23.6216) (-37.8676, 23.6301) (-37.8223, 23.6384) (-37.7768, 23.6464) (-37.7312, 23.6542) (-37.6854, 23.6617) (-37.6396, 23.669) (-37.5935, 23.676) (-37.5474, 23.6827) (-37.5104, 23.6879) (-37.4826, 23.6917) (-37.464, 23.6942) (-37.4547, 23.6954) knots 0 0 0 0 0 0 0.01428571 0.02857143 0.04285714 0.05714286 0.07142857 0.08571429 0.1 0.11428571 0.12857143 0.14285714 0.15714286 0.17142857 0.18571429 0.2 0.21428571 0.22857143 0.24285714 0.25714286 0.27142857 0.28571429 0.3 0.31428571 0.32857143 0.34285714 0.35714286 0.37142857 0.38571429 0.4 0.41428571 0.42857143 0.44285714 0.45714286 0.47142857 0.48571429 0.5 0.51428571 0.52857143 0.54285714 0.55714286 0.57142857 0.58571429 0.6 0.61428571 0.62857143 0.64285714 0.65714286 0.67142857 0.68571429 0.7 0.71428571 0.72857143 0.74285714 0.75714286 0.77142857 0.78571429 0.8 0.81428571 0.82857143 0.84285714 0.85714286 0.87142857 0.88571429 0.9 0.91428571 0.92857143 0.94285714 0.95714286 0.97142857 0.98571429 1 1 1 1 1 1
  line L9 (-40.2516, 22.5911) -> (-41.0866, 21.6088)
  arc A19 (-41.7716, 21.5356) -> (-41.0866, 21.6088) centre (-41.4675, 21.9326) ccw
  arc A20 (-41.7716, 21.5356) -> (-42.8124, 22.229) centre (-47.5478, 13.9934) ccw
  arc A21 (-43.0087, 22.8893) -> (-42.8124, 22.229) centre (-42.5631, 22.6625) ccw
  line L10 (-43.0087, 22.8893) -> (-42.4238, 24.0383)
  spline S10 degree 5 poles (-42.4238, 24.0383) (-42.4201, 24.0455) (-42.413, 24.06) (-42.4031, 24.0821) (-42.3911, 24.112) (-42.3781, 24.1503) (-42.3663, 24.1892) (-42.3553, 24.2284) (-42.3448, 24.2678) (-42.3346, 24.3074) (-42.3247, 24.3471) (-42.3153, 24.387) (-42.3064, 24.4271) (-42.2982, 24.4675) (-42.2906, 24.5082) (-42.2836, 24.5491) (-42.2772, 24.5902) (-42.2712, 24.6314) (-42.2657, 24.6728) (-42.2604, 24.7143) (-42.2556, 24.756) (-42.2512, 24.7978) (-42.2471, 24.8398) (-42.2435, 24.8818) (-42.2404, 24.9241) (-42.2376, 24.9664) (-42.2352, 25.0089) (-42.2332, 25.0515) (-42.2316, 25.0942) (-42.2303, 25.1371) (-42.2294, 25.18) (-42.2288, 25.223) (-42.2286, 25.2661) (-42.2287, 25.3094) (-42.2292, 25.3527) (-42.2301, 25.3961) (-42.2313, 25.4396) (-42.2328, 25.4832) (-42.2346, 25.5268) (-42.2368, 25.5706) (-42.2393, 25.6144) (-42.2422, 25.6583) (-42.2453, 25.7022) (-42.2488, 25.7463) (-42.2526, 25.7904) (-42.2567, 25.8345) (-42.2612, 25.8788) (-42.2659, 25.9231) (-42.271, 25.9674) (-42.2764, 26.0118) (-42.282, 26.0563) (-42.288, 26.1008) (-42.2943, 26.1454) (-42.3009, 26.19) (-42.3078, 26.2347) (-42.315, 26.2794) (-42.3225, 26.3241) (-42.3303, 26.3689) (-42.3383, 26.4138) (-42.3467, 26.4586) (-42.3554, 26.5035) (-42.3643, 26.5485) (-42.3736, 26.5935) (-42.3831, 26.6385) (-42.393, 26.6835) (-42.4031, 26.7286) (-42.4135, 26.7737) (-42.4242, 26.8188) (-42.4351, 26.8639) (-42.4464, 26.9091) (-42.4579, 26.9543) (-42.4674, 26.9904) (-42.4746, 27.0176) (-42.4794, 27.0357) (-42.4819, 27.0447) knots 0 0 0 0 0 0 0.01428571 0.02857143 0.04285714 0.05714286 0.07142857 0.08571429 0.1 0.11428571 0.12857143 0.14285714 0.15714286 0.17142857 0.18571429 0.2 0.21428571 0.22857143 0.24285714 0.25714286 0.27142857 0.28571429 0.3 0.31428571 0.32857143 0.34285714 0.35714286 0.37142857 0.38571429 0.4 0.41428571 0.42857143 0.44285714 0.45714286 0.47142857 0.48571429 0.5 0.51428571 0.52857143 0.54285714 0.55714286 0.57142857 0.58571429 0.6 0.61428571 0.62857143 0.64285714 0.65714286 0.67142857 0.68571429 0.7 0.71428571 0.72857143 0.74285714 0.75714286 0.77142857 0.78571429 0.8 0.81428571 0.82857143 0.84285714 0.85714286 0.87142857 0.88571429 0.9 0.91428571 0.92857143 0.94285714 0.95714286 0.97142857 0.98571429 1 1 1 1 1 1
  arc A22 (-42.4819, 27.0447) -> (-43.6579, 27.4422) centre (-47.5478, 13.9934) ccw
  spline S11 degree 5 poles (-45.5279, 25.0873) (-45.5265, 25.0953) (-45.5233, 25.1111) (-45.5178, 25.1347) (-45.5091, 25.1658) (-45.4963, 25.2041) (-45.4821, 25.2422) (-45.467, 25.28) (-45.4515, 25.3177) (-45.4356, 25.3554) (-45.4193, 25.3929) (-45.4026, 25.4304) (-45.3854, 25.4677) (-45.3674, 25.5048) (-45.3487, 25.5417) (-45.3295, 25.5784) (-45.3097, 25.615) (-45.2894, 25.6514) (-45.2687, 25.6877) (-45.2477, 25.7239) (-45.2262, 25.76) (-45.2044, 25.7959) (-45.1822, 25.8317) (-45.1595, 25.8673) (-45.1364, 25.9028) (-45.1129, 25.9382) (-45.089, 25.9734) (-45.0647, 26.0085) (-45.0401, 26.0434) (-45.0152, 26.0782) (-44.9899, 26.1129) (-44.9642, 26.1475) (-44.9382, 26.1819) (-44.9119, 26.2161) (-44.8852, 26.2503) (-44.8582, 26.2843) (-44.8309, 26.3181) (-44.8033, 26.3519) (-44.7753, 26.3855) (-44.747, 26.4189) (-44.7185, 26.4522) (-44.6896, 26.4854) (-44.6604, 26.5184) (-44.6309, 26.5513) (-44.6011, 26.5841) (-44.5711, 26.6167) (-44.5407, 26.6492) (-44.5101, 26.6815) (-44.4791, 26.7137) (-44.4479, 26.7457) (-44.4164, 26.7776) (-44.3847, 26.8094) (-44.3526, 26.841) (-44.3203, 26.8725) (-44.2878, 26.9038) (-44.2549, 26.935) (-44.2218, 26.966) (-44.1884, 26.9969) (-44.1548, 27.0276) (-44.1209, 27.0582) (-44.0868, 27.0887) (-44.0524, 27.119) (-44.0178, 27.1491) (-43.9829, 27.1791) (-43.9477, 27.209) (-43.9124, 27.2387) (-43.8767, 27.2682) (-43.8409, 27.2976) (-43.8048, 27.3268) (-43.7684, 27.3559) (-43.7319, 27.3848) (-43.7024, 27.4078) (-43.6802, 27.425) (-43.6654, 27.4365) (-43.6579, 27.4422) knots 0 0 0 0 0 0 0.01428571 0.02857143 0.04285714 0.05714286 0.07142857 0.08571429 0.1 0.11428571 0.12857143 0.14285714 0.15714286 0.17142857 0.18571429 0.2 0.21428571 0.22857143 0.24285714 0.25714286 0.27142857 0.28571429 0.3 0.31428571 0.32857143 0.34285714 0.35714286 0.37142857 0.38571429 0.4 0.41428571 0.42857143 0.44285714 0.45714286 0.47142857 0.48571429 0.5 0.51428571 0.52857143 0.54285714 0.55714286 0.57142857 0.58571429 0.6 0.61428571 0.62857143 0.64285714 0.65714286 0.67142857 0.68571429 0.7 0.71428571 0.72857143 0.74285714 0.75714286 0.77142857 0.78571429 0.8 0.81428571 0.82857143 0.84285714 0.85714286 0.87142857 0.88571429 0.9 0.91428571 0.92857143 0.94285714 0.95714286 0.97142857 0.98571429 1 1 1 1 1 1
  line L11 (-45.5279, 25.0873) -> (-45.7599, 23.8191)
  arc A23 (-46.3165, 23.4133) -> (-45.7599, 23.8191) centre (-46.2517, 23.9091) ccw
  arc A24 (-46.3165, 23.4133) -> (-47.5646, 23.4934) centre (-47.5478, 13.9934) ccw
  arc A25 (-48.0648, 23.9671) -> (-47.5646, 23.4934) centre (-47.5655, 23.9934) ccw
  line L12 (-48.0648, 23.9671) -> (-48.1327, 25.2546)
  spline S12 degree 5 poles (-48.1327, 25.2546) (-48.1331, 25.2626) (-48.1342, 25.2787) (-48.1366, 25.3028) (-48.1413, 25.3347) (-48.1491, 25.3744) (-48.1584, 25.414) (-48.1685, 25.4534) (-48.1791, 25.4928) (-48.19, 25.5322) (-48.2013, 25.5715) (-48.2131, 25.6108) (-48.2255, 25.65) (-48.2385, 25.6891) (-48.2523, 25.7281) (-48.2667, 25.767) (-48.2817, 25.8058) (-48.2972, 25.8445) (-48.313, 25.8831) (-48.3293, 25.9217) (-48.3459, 25.9602) (-48.363, 25.9986) (-48.3805, 26.037) (-48.3984, 26.0752) (-48.4168, 26.1134) (-48.4355, 26.1514) (-48.4547, 26.1894) (-48.4743, 26.2273) (-48.4942, 26.2651) (-48.5145, 26.3029) (-48.5352, 26.3405) (-48.5562, 26.378) (-48.5776, 26.4155) (-48.5993, 26.4528) (-48.6214, 26.4901) (-48.6439, 26.5273) (-48.6666, 26.5644) (-48.6897, 26.6013) (-48.7132, 26.6382) (-48.7369, 26.675) (-48.761, 26.7117) (-48.7854, 26.7483) (-48.8101, 26.7848) (-48.8352, 26.8212) (-48.8605, 26.8575) (-48.8862, 26.8937) (-48.9121, 26.9298) (-48.9384, 26.9658) (-48.9649, 27.0016) (-48.9918, 27.0374) (-49.019, 27.0731) (-49.0464, 27.1086) (-49.0741, 27.1441) (-49.1021, 27.1794) (-49.1304, 27.2147) (-49.159, 27.2498) (-49.1879, 27.2848) (-49.217, 27.3197) (-49.2464, 27.3545) (-49.2761, 27.3892) (-49.3061, 27.4237) (-49.3363, 27.4582) (-49.3668, 27.4925) (-49.3976, 27.5267) (-49.4286, 27.5608) (-49.4599, 27.5948) (-49.4915, 27.6286) (-49.5233, 27.6624) (-49.5554, 27.696) (-49.5877, 27.7294) (-49.6203, 27.7628) (-49.6465, 27.7894) (-49.6663, 27.8093) (-49.6796, 27.8225) (-49.6862, 27.8291) knots 0 0 0 0 0 0 0.01428571 0.02857143 0.04285714 0.05714286 0.07142857 0.08571429 0.1 0.11428571 0.12857143 0.14285714 0.15714286 0.17142857 0.18571429 0.2 0.21428571 0.22857143 0.24285714 0.25714286 0.27142857 0.28571429 0.3 0.31428571 0.32857143 0.34285714 0.35714286 0.37142857 0.38571429 0.4 0.41428571 0.42857143 0.44285714 0.45714286 0.47142857 0.48571429 0.5 0.51428571 0.52857143 0.54285714 0.55714286 0.57142857 0.58571429 0.6 0.61428571 0.62857143 0.64285714 0.65714286 0.67142857 0.68571429 0.7 0.71428571 0.72857143 0.74285714 0.75714286 0.77142857 0.78571429 0.8 0.81428571 0.82857143 0.84285714 0.85714286 0.87142857 0.88571429 0.9 0.91428571 0.92857143 0.94285714 0.95714286 0.97142857 0.98571429 1 1 1 1 1 1
  arc A26 (-49.6862, 27.8291) -> (-50.9035, 27.5853) centre (-47.5478, 13.9934) ccw
  spline S13 degree 5 poles (-51.3455, 24.611) (-51.3482, 24.6186) (-51.3534, 24.6339) (-51.3604, 24.657) (-51.3684, 24.6883) (-51.3765, 24.7279) (-51.3832, 24.768) (-51.3891, 24.8083) (-51.3945, 24.8487) (-51.3995, 24.8893) (-51.4043, 24.9299) (-51.4085, 24.9707) (-51.4122, 25.0117) (-51.4152, 25.0528) (-51.4175, 25.0941) (-51.4192, 25.1355) (-51.4203, 25.1771) (-51.4209, 25.2188) (-51.4212, 25.2605) (-51.4211, 25.3024) (-51.4205, 25.3443) (-51.4196, 25.3864) (-51.4182, 25.4285) (-51.4164, 25.4707) (-51.4142, 25.513) (-51.4115, 25.5553) (-51.4084, 25.5978) (-51.4049, 25.6403) (-51.4011, 25.6829) (-51.3969, 25.7255) (-51.3923, 25.7682) (-51.3874, 25.8109) (-51.3821, 25.8537) (-51.3764, 25.8966) (-51.3704, 25.9395) (-51.364, 25.9824) (-51.3573, 26.0254) (-51.3502, 26.0684) (-51.3428, 26.1115) (-51.335, 26.1546) (-51.3269, 26.1977) (-51.3185, 26.2409) (-51.3097, 26.2841) (-51.3006, 26.3273) (-51.2912, 26.3706) (-51.2815, 26.4139) (-51.2714, 26.4572) (-51.2611, 26.5005) (-51.2504, 26.5438) (-51.2394, 26.5872) (-51.2281, 26.6306) (-51.2164, 26.674) (-51.2045, 26.7174) (-51.1923, 26.7608) (-51.1797, 26.8042) (-51.1669, 26.8476) (-51.1537, 26.891) (-51.1403, 26.9345) (-51.1265, 26.9779) (-51.1125, 27.0213) (-51.0981, 27.0648) (-51.0835, 27.1082) (-51.0686, 27.1516) (-51.0533, 27.195) (-51.0378, 27.2385) (-51.022, 27.2819) (-51.006, 27.3253) (-50.9896, 27.3686) (-50.9729, 27.412) (-50.956, 27.4554) (-50.9388, 27.4987) (-50.9248, 27.5334) (-50.9142, 27.5593) (-50.907, 27.5767) (-50.9035, 27.5853) knots 0 0 0 0 0 0 0.01428571 0.02857143 0.04285714 0.05714286 0.07142857 0.08571429 0.1 0.11428571 0.12857143 0.14285714 0.15714286 0.17142857 0.18571429 0.2 0.21428571 0.22857143 0.24285714 0.25714286 0.27142857 0.28571429 0.3 0.31428571 0.32857143 0.34285714 0.35714286 0.37142857 0.38571429 0.4 0.41428571 0.42857143 0.44285714 0.45714286 0.47142857 0.48571429 0.5 0.51428571 0.52857143 0.54285714 0.55714286 0.57142857 0.58571429 0.6 0.61428571 0.62857143 0.64285714 0.65714286 0.67142857 0.68571429 0.7 0.71428571 0.72857143 0.74285714 0.75714286 0.77142857 0.78571429 0.8 0.81428571 0.82857143 0.84285714 0.85714286 0.87142857 0.88571429 0.9 0.91428571 0.92857143 0.94285714 0.95714286 0.97142857 0.98571429 1 1 1 1 1 1
  line L13 (-51.3455, 24.611) -> (-50.9123, 23.3967)
  arc A27 (-51.1914, 22.7669) -> (-50.9123, 23.3967) centre (-51.3832, 23.2287) ccw
  arc A28 (-51.1914, 22.7669) -> (-52.3123, 22.2123) centre (-47.5478, 13.9934) ccw
  arc A29 (-52.9824, 22.3724) -> (-52.3123, 22.2123) centre (-52.5631, 22.6448) ccw
  line L14 (-52.9824, 22.3724) -> (-53.6849, 23.4534)
  spline S14 degree 5 poles (-53.6849, 23.4534) (-53.6893, 23.4602) (-53.6983, 23.4736) (-53.7125, 23.4932) (-53.7325, 23.5186) (-53.7591, 23.549) (-53.7868, 23.5786) (-53.8153, 23.6077) (-53.8442, 23.6365) (-53.8734, 23.6652) (-53.9028, 23.6936) (-53.9326, 23.7217) (-53.963, 23.7495) (-53.9938, 23.7768) (-54.0253, 23.8037) (-54.0572, 23.8302) (-54.0896, 23.8563) (-54.1223, 23.8821) (-54.1554, 23.9076) (-54.1887, 23.9329) (-54.2224, 23.9579) (-54.2564, 23.9827) (-54.2907, 24.0071) (-54.3253, 24.0313) (-54.3603, 24.0552) (-54.3956, 24.0787) (-54.4312, 24.102) (-54.4671, 24.1251) (-54.5033, 24.1478) (-54.5397, 24.1703) (-54.5765, 24.1926) (-54.6134, 24.2146) (-54.6507, 24.2364) (-54.6882, 24.2578) (-54.7259, 24.2791) (-54.7639, 24.3001) (-54.8022, 24.3208) (-54.8407, 24.3413) (-54.8794, 24.3615) (-54.9184, 24.3815) (-54.9576, 24.4012) (-54.9971, 24.4207) (-55.0367, 24.4399) (-55.0766, 24.4589) (-55.1167, 24.4777) (-55.157, 24.4962) (-55.1975, 24.5145) (-55.2383, 24.5325) (-55.2792, 24.5503) (-55.3203, 24.5679) (-55.3617, 24.5852) (-55.4032, 24.6023) (-55.445, 24.6191) (-55.4869, 24.6357) (-55.529, 24.6521) (-55.5713, 24.6682) (-55.6139, 24.6841) (-55.6565, 24.6997) (-55.6994, 24.7151) (-55.7425, 24.7303) (-55.7857, 24.7453) (-55.8291, 24.76) (-55.8727, 24.7745) (-55.9164, 24.7887) (-55.9603, 24.8027) (-56.0044, 24.8165) (-56.0487, 24.83) (-56.0931, 24.8433) (-56.1377, 24.8564) (-56.1824, 24.8692) (-56.2273, 24.8818) (-56.2633, 24.8917) (-56.2905, 24.8991) (-56.3086, 24.9039) (-56.3176, 24.9063) knots 0 0 0 0 0 0 0.01428571 0.02857143 0.04285714 0.05714286 0.07142857 0.08571429 0.1 0.11428571 0.12857143 0.14285714 0.15714286 0.17142857 0.18571429 0.2 0.21428571 0.22857143 0.24285714 0.25714286 0.27142857 0.28571429 0.3 0.31428571 0.32857143 0.34285714 0.35714286 0.37142857 0.38571429 0.4 0.41428571 0.42857143 0.44285714 0.45714286 0.47142857 0.48571429 0.5 0.51428571 0.52857143 0.54285714 0.55714286 0.57142857 0.58571429 0.6 0.61428571 0.62857143 0.64285714 0.65714286 0.67142857 0.68571429 0.7 0.71428571 0.72857143 0.74285714 0.75714286 0.77142857 0.78571429 0.8 0.81428571 0.82857143 0.84285714 0.85714286 0.87142857 0.88571429 0.9 0.91428571 0.92857143 0.94285714 0.95714286 0.97142857 0.98571429 1 1 1 1 1 1
  arc A30 (-56.3176, 24.9063) -> (-57.2498, 24.0865) centre (-47.5478, 13.9934) ccw
  spline S15 degree 5 poles (-56.1455, 21.2897) (-56.1517, 21.2949) (-56.1638, 21.3056) (-56.1815, 21.3221) (-56.204, 21.3452) (-56.2308, 21.3754) (-56.2567, 21.4068) (-56.2819, 21.4387) (-56.3068, 21.4711) (-56.3314, 21.5037) (-56.3558, 21.5365) (-56.3799, 21.5697) (-56.4036, 21.6033) (-56.4267, 21.6374) (-56.4494, 21.672) (-56.4715, 21.7071) (-56.4933, 21.7425) (-56.5147, 21.7783) (-56.5358, 21.8143) (-56.5566, 21.8507) (-56.5771, 21.8872) (-56.5973, 21.9241) (-56.6172, 21.9613) (-56.6367, 21.9987) (-56.6559, 22.0365) (-56.6748, 22.0745) (-56.6934, 22.1128) (-56.7116, 22.1514) (-56.7296, 22.1901) (-56.7472, 22.2292) (-56.7646, 22.2684) (-56.7817, 22.3079) (-56.7985, 22.3476) (-56.815, 22.3876) (-56.8313, 22.4277) (-56.8472, 22.4681) (-56.8629, 22.5087) (-56.8783, 22.5495) (-56.8934, 22.5905) (-56.9082, 22.6317) (-56.9228, 22.6731) (-56.9371, 22.7147) (-56.9511, 22.7565) (-56.9648, 22.7985) (-56.9783, 22.8407) (-56.9915, 22.883) (-57.0044, 22.9255) (-57.0171, 22.9682) (-57.0295, 23.0111) (-57.0417, 23.0542) (-57.0536, 23.0974) (-57.0652, 23.1408) (-57.0766, 23.1843) (-57.0877, 23.228) (-57.0985, 23.2719) (-57.1091, 23.316) (-57.1194, 23.3601) (-57.1295, 23.4045) (-57.1393, 23.449) (-57.1488, 23.4936) (-57.1581, 23.5384) (-57.1672, 23.5833) (-57.176, 23.6284) (-57.1845, 23.6736) (-57.1928, 23.719) (-57.2008, 23.7644) (-57.2086, 23.8101) (-57.2161, 23.8558) (-57.2234, 23.9017) (-57.2304, 23.9477) (-57.2371, 23.9938) (-57.2423, 24.0309) (-57.2461, 24.0587) (-57.2486, 24.0772) (-57.2498, 24.0865) knots 0 0 0 0 0 0 0.01428571 0.02857143 0.04285714 0.05714286 0.07142857 0.08571429 0.1 0.11428571 0.12857143 0.14285714 0.15714286 0.17142857 0.18571429 0.2 0.21428571 0.22857143 0.24285714 0.25714286 0.27142857 0.28571429 0.3 0.31428571 0.32857143 0.34285714 0.35714286 0.37142857 0.38571429 0.4 0.41428571 0.42857143 0.44285714 0.45714286 0.47142857 0.48571429 0.5 0.51428571 0.52857143 0.54285714 0.55714286 0.57142857 0.58571429 0.6 0.61428571 0.62857143 0.64285714 0.65714286 0.67142857 0.68571429 0.7 0.71428571 0.72857143 0.74285714 0.75714286 0.77142857 0.78571429 0.8 0.81428571 0.82857143 0.84285714 0.85714286 0.87142857 0.88571429 0.9 0.91428571 0.92857143 0.94285714 0.95714286 0.97142857 0.98571429 1 1 1 1 1 1
  line L15 (-56.1455, 21.2897) -> (-55.1632, 20.4547)
  arc A31 (-55.09, 19.7697) -> (-55.1632, 20.4547) centre (-55.487, 20.0737) ccw
  arc A32 (-55.09, 19.7697) -> (-55.7834, 18.7289) centre (-47.5478, 13.9934) ccw
  arc A33 (-56.4437, 18.5325) -> (-55.7834, 18.7289) centre (-56.2169, 18.9781) ccw
  line L16 (-56.4437, 18.5325) -> (-57.5927, 19.1175)
  spline S16 degree 5 poles (-57.5927, 19.1175) (-57.5999, 19.1211) (-57.6144, 19.1282) (-57.6365, 19.1382) (-57.6664, 19.1501) (-57.7047, 19.1632) (-57.7436, 19.175) (-57.7828, 19.1859) (-57.8222, 19.1964) (-57.8618, 19.2066) (-57.9015, 19.2165) (-57.9414, 19.226) (-57.9815, 19.2349) (-58.0219, 19.2431) (-58.0626, 19.2506) (-58.1035, 19.2576) (-58.1446, 19.264) (-58.1858, 19.27) (-58.2272, 19.2756) (-58.2687, 19.2808) (-58.3104, 19.2857) (-58.3522, 19.2901) (-58.3942, 19.2941) (-58.4362, 19.2977) (-58.4785, 19.3009) (-58.5208, 19.3037) (-58.5633, 19.306) (-58.6059, 19.308) (-58.6487, 19.3097) (-58.6915, 19.3109) (-58.7344, 19.3119) (-58.7774, 19.3124) (-58.8205, 19.3126) (-58.8638, 19.3125) (-58.9071, 19.312) (-58.9505, 19.3112) (-58.994, 19.31) (-59.0376, 19.3085) (-59.0812, 19.3066) (-59.125, 19.3044) (-59.1688, 19.3019) (-59.2127, 19.2991) (-59.2566, 19.2959) (-59.3007, 19.2924) (-59.3448, 19.2886) (-59.3889, 19.2845) (-59.4332, 19.2801) (-59.4775, 19.2753) (-59.5218, 19.2703) (-59.5662, 19.2649) (-59.6107, 19.2592) (-59.6552, 19.2532) (-59.6998, 19.2469) (-59.7444, 19.2404) (-59.7891, 19.2335) (-59.8338, 19.2263) (-59.8785, 19.2188) (-59.9233, 19.211) (-59.9682, 19.2029) (-60.013, 19.1945) (-60.0579, 19.1859) (-60.1029, 19.1769) (-60.1479, 19.1677) (-60.1929, 19.1581) (-60.2379, 19.1483) (-60.283, 19.1382) (-60.3281, 19.1278) (-60.3732, 19.1171) (-60.4183, 19.1061) (-60.4635, 19.0949) (-60.5087, 19.0833) (-60.5449, 19.0739) (-60.572, 19.0667) (-60.5901, 19.0618) (-60.5991, 19.0594) knots 0 0 0 0 0 0 0.01428571 0.02857143 0.04285714 0.05714286 0.07142857 0.08571429 0.1 0.11428571 0.12857143 0.14285714 0.15714286 0.17142857 0.18571429 0.2 0.21428571 0.22857143 0.24285714 0.25714286 0.27142857 0.28571429 0.3 0.31428571 0.32857143 0.34285714 0.35714286 0.37142857 0.38571429 0.4 0.41428571 0.42857143 0.44285714 0.45714286 0.47142857 0.48571429 0.5 0.51428571 0.52857143 0.54285714 0.55714286 0.57142857 0.58571429 0.6 0.61428571 0.62857143 0.64285714 0.65714286 0.67142857 0.68571429 0.7 0.71428571 0.72857143 0.74285714 0.75714286 0.77142857 0.78571429 0.8 0.81428571 0.82857143 0.84285714 0.85714286 0.87142857 0.88571429 0.9 0.91428571 0.92857143 0.94285714 0.95714286 0.97142857 0.98571429 1 1 1 1 1 1
  arc A34 (-60.5991, 19.0594) -> (-60.9966, 17.8833) centre (-47.5478, 13.9934) ccw